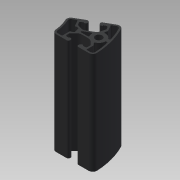
# Autodesk Inventor part: 40-4093-BLACK-FB
Saved by Autodesk Inventor 2013 (Build 170138000, 138)
## iProperties
Company: 80/20 Inc.
Created: 2014-04-23
Part Number: 40-4093-BLACK-FB
Material: Generic
Document SubType Name: Modeling
Designer: Ross Bowman
Density: 1 g/cm^3
Engineer: Ross Bowman
Catalog Web Link: 8020.net
Vendor: 80/20 Inc.
Material: 6105-T5 Aluminum
Author: Ross Bowman
Keywords: 80/20 , 8020 , T-Slot , Extrusion
Autodesk Inventor part; units mm, degrees
ref_plane "YZ Plane" through (0, 0, 0) normal (1, 0, 0) x (0, 1, 0)
ref_plane "XZ Plane" through (0, 0, 0) normal (0, 1, 0) x (-1, 0, 0)
ref_plane "XY Plane" through (0, 0, 0) normal (0, 0, 1) x (1, 0, 0)
sketch "Sketch1" plane through (0, 0, 0) normal (0, 0, 1) x (1, 0, 0)
  circle A0 centre (0, 0) radius 3.4
  arc A1 (-6.641, -0.198) -> (-5.8503, -3.149) centre (0, 0) ccw
  arc A2 (-6.5195, -4.2692) -> (-5.8503, -3.149) centre (-6.5195, -3.5092) ccw
  line L0 (-13.0965, -4.2692) -> (-6.5195, -4.2692)
  arc A3 (-13.4765, -2.851) -> (-13.0965, -4.2692) centre (-13.0965, -3.5092) ccw
  line L1 (-7.7807, 0.4375) -> (-13.4765, -2.851)
  arc A4 (-6.641, -0.198) -> (-7.7807, 0.4375) centre (-7.4007, -0.2207) ccw
  arc A5 (-1.5101, 7.5599) -> (-0.6963, 6.6074) centre (-0.776, 7.3632) ccw
  line L2 (-0.9407, 9.685) -> (-1.5101, 7.5599)
  arc A6 (-0.9407, 9.685) -> (-1.0166, 10.2617) centre (-1.6748, 9.8817) ccw
  line L3 (-4.1504, 15.6896) -> (-1.0166, 10.2617)
  arc A7 (-3.8793, 16.7237) -> (-4.1504, 15.6896) centre (-3.4922, 16.0696) ccw
  line L4 (-1.0754, 18.3829) -> (-3.8793, 16.7237)
  arc A8 (2.2157, 17.4265) -> (-1.0754, 18.3829) centre (0.1214, 16.3605) ccw
  arc A9 (7.4116, 4.4816) -> (2.2157, 17.4265) centre (-67.6148, -18.1173) ccw
  arc A10 (6.8805, 3.5283) -> (7.4116, 4.4816) centre (6.6838, 4.2624) ccw
  line L5 (6.3485, 3.3858) -> (6.8805, 3.5283)
  arc A11 (5.5204, 3.697) -> (6.3485, 3.3858) centre (6.1518, 4.1199) ccw
  arc A12 (5.5204, 3.697) -> (-0.6963, 6.6074) centre (0, 0) ccw
  arc A13 (2.7006, -6.0703) -> (6.6293, -0.4415) centre (0, 0) ccw
  arc A14 (7.1909, 0.2421) -> (6.6293, -0.4415) centre (7.3876, -0.492) ccw
  line L6 (7.7229, 0.3846) -> (7.1909, 0.2421)
  arc A15 (8.6594, -0.1754) -> (7.7229, 0.3846) centre (7.9196, -0.3495) ccw
  arc A16 (10.6314, -13.97) -> (8.6594, -0.1754) centre (-67.6148, -18.1173) ccw
  line L7 (4.2504, -9.3952) -> (4.2504, -15.6844)
  arc A17 (4.2504, -9.3952) -> (4.0278, -8.8578) centre (3.4904, -9.3952) ccw
  line L8 (2.4722, -7.3021) -> (4.0278, -8.8578)
  arc A18 (2.7006, -6.0703) -> (2.4722, -7.3021) centre (3.0096, -6.7647) ccw
  arc A19 (-17.472, -2.5855) -> (-17.8859, -2.093) centre (-18.2061, -2.7822) ccw
  line L9 (-16.4239, -6.4969) -> (-17.472, -2.5855)
  arc A20 (-16.5361, -7.1304) -> (-16.4239, -6.4969) centre (-17.158, -6.6936) ccw
  arc A21 (-18.8445, -8.5432) -> (-16.5361, -7.1304) centre (-19.3185, -5.1764) ccw
  arc A22 (-18.8445, -8.5432) -> (-19.4985, -9.2957) centre (-18.7385, -9.2957) ccw
  line L10 (-19.4985, -15.6844) -> (-19.4985, -9.2957)
  arc A23 (-26.1453, -14.3093) -> (-29.8036, -0.6665) centre (-67.6148, -18.1173) ccw
  arc A24 (-28.8231, 2.3659) -> (-29.8036, -0.6665) centre (-27.6699, 0.3183) ccw
  line L11 (-25.7487, 4.0973) -> (-28.8231, 2.3659)
  arc A25 (-24.7176, 3.8151) -> (-25.7487, 4.0973) centre (-25.3758, 3.4351) ccw
  line L12 (-21.5341, -1.6989) -> (-24.7176, 3.8151)
  arc A26 (-21.5341, -1.6989) -> (-20.5914, -2.0236) centre (-20.8759, -1.3189) ccw
  arc A27 (-17.8859, -2.093) -> (-20.5914, -2.0236) centre (-19.3185, -5.1764) ccw
  arc A28 (-3.5707, -16.5209) -> (-2.0596, -18.1044) centre (-1.9773, -16.5131) ccw
  line L13 (-2.0596, -18.1044) -> (8.2792, -18.1044)
  arc A29 (8.2792, -18.1044) -> (12.2736, -13.8932) centre (8.2792, -14.1044) ccw
  arc A30 (12.2736, -13.8932) -> (3.6826, 18.1687) centre (-67.6148, -18.1173) ccw
  arc A31 (3.6826, 18.1687) -> (-1.8822, 19.8185) centre (0.1178, 16.3544) ccw
  line L14 (-1.8822, 19.8185) -> (-10.8359, 14.6491)
  arc A32 (-10.8359, 14.6491) -> (-11.3528, 12.5222) centre (-9.969, 13.3121) ccw
  line L15 (-11.3528, 12.5222) -> (-10.8956, 11.7304)
  arc A33 (-10.8956, 11.7304) -> (-8.8041, 11.13) centre (-9.5411, 12.5058) ccw
  line L16 (-8.8041, 11.13) -> (-8.1373, 11.515)
  arc A34 (-8.1373, 11.515) -> (-7.9918, 12.0224) centre (-8.3273, 11.844) ccw
  line L17 (-7.9918, 12.0224) -> (-8.0052, 12.0476)
  arc A35 (-7.8597, 12.555) -> (-8.0052, 12.0476) centre (-7.6697, 12.226) ccw
  line L18 (-7.8597, 12.555) -> (-6.2048, 13.5105)
  arc A36 (-4.4702, 13.0457) -> (-6.2048, 13.5105) centre (-5.5699, 12.4107) ccw
  line L19 (-4.4702, 13.0457) -> (-3.2502, 10.9325)
  arc A37 (-3.1614, 10.258) -> (-3.2502, 10.9325) centre (-4.02, 10.488) ccw
  line L20 (-3.1614, 10.258) -> (-4.3643, 5.7687)
  arc A38 (-6.577, 2.8849) -> (-4.3643, 5.7687) centre (-8.9516, 6.9979) ccw
  line L21 (-6.577, 2.8849) -> (-12.4327, -0.4958)
  arc A39 (-16.0365, -0.9703) -> (-12.4327, -0.4958) centre (-14.8073, 3.6171) ccw
  line L22 (-16.0365, -0.9703) -> (-20.5258, 0.2326)
  arc A40 (-21.0655, 0.6468) -> (-20.5258, 0.2326) centre (-20.2957, 1.0912) ccw
  line L23 (-21.0655, 0.6468) -> (-22.2856, 2.76)
  arc A41 (-21.8208, 4.4946) -> (-22.2856, 2.76) centre (-21.1859, 3.3949) ccw
  line L24 (-21.8208, 4.4946) -> (-20.1659, 5.45)
  arc A42 (-19.6537, 5.3223) -> (-20.1659, 5.45) centre (-19.976, 5.121) ccw
  line L25 (-19.6537, 5.3223) -> (-19.6386, 5.2981)
  arc A43 (-19.6386, 5.2981) -> (-19.1264, 5.1704) centre (-19.3164, 5.4995) ccw
  line L26 (-19.1264, 5.1704) -> (-18.5146, 5.5237)
  arc A44 (-18.5146, 5.5237) -> (-17.9383, 7.6746) centre (-19.3019, 6.8873) ccw
  line L27 (-17.9383, 7.6746) -> (-18.3954, 8.4664)
  arc A45 (-18.3954, 8.4664) -> (-20.5464, 9.0427) centre (-19.759, 7.6791) ccw
  line L28 (-20.5464, 9.0427) -> (-29.662, 3.7798)
  arc A46 (-29.662, 3.7798) -> (-31.2941, -1.36) centre (-27.662, 0.3157) ccw
  arc A47 (-27.7815, -14.4692) -> (-31.2941, -1.36) centre (-67.6148, -18.1173) ccw
  arc A48 (-27.7815, -14.4692) -> (-23.7982, -18.1044) centre (-23.7982, -14.1044) ccw
  line L29 (-23.7982, -18.1044) -> (-13.2723, -18.1044)
  arc A49 (-13.2723, -18.1044) -> (-11.6977, -16.5298) centre (-13.2723, -16.5298) ccw
  line L30 (-11.6977, -16.5298) -> (-11.6977, -15.6155)
  arc A50 (-11.6977, -15.6155) -> (-13.2723, -14.0409) centre (-13.2723, -15.6155) ccw
  line L31 (-13.2723, -14.0409) -> (-13.9788, -14.0409)
  arc A51 (-13.9788, -14.0409) -> (-14.3585, -14.4076) centre (-13.9788, -14.4209) ccw
  line L32 (-14.3585, -14.4076) -> (-14.3595, -14.4361)
  arc A52 (-14.7392, -14.8028) -> (-14.3595, -14.4361) centre (-14.7392, -14.4229) ccw
  line L33 (-14.7392, -14.8028) -> (-16.6501, -14.8028)
  arc A53 (-17.9199, -13.533) -> (-16.6501, -14.8028) centre (-16.6501, -13.533) ccw
  line L34 (-17.9199, -13.533) -> (-17.9199, -11.0929)
  arc A54 (-17.6596, -10.4644) -> (-17.9199, -11.0929) centre (-17.031, -11.0929) ccw
  line L35 (-17.6596, -10.4644) -> (-14.3732, -7.178)
  arc A55 (-11.015, -5.787) -> (-14.3732, -7.178) centre (-11.015, -10.5362) ccw
  line L36 (-11.015, -5.787) -> (-4.2534, -5.787)
  arc A56 (-0.8952, -7.178) -> (-4.2534, -5.787) centre (-4.2534, -10.5362) ccw
  line L37 (-0.8952, -7.178) -> (2.3912, -10.4644)
  arc A57 (2.6515, -11.0929) -> (2.3912, -10.4644) centre (1.7626, -11.0929) ccw
  line L38 (2.6515, -11.0929) -> (2.6515, -13.533)
  arc A58 (1.3817, -14.8028) -> (2.6515, -13.533) centre (1.3817, -13.533) ccw
  line L39 (1.3817, -14.8028) -> (-0.5292, -14.8028)
  arc A59 (-0.9089, -14.4361) -> (-0.5292, -14.8028) centre (-0.5292, -14.4229) ccw
  line L40 (-0.9089, -14.4361) -> (-0.9099, -14.4076)
  arc A60 (-0.9099, -14.4076) -> (-1.2896, -14.0409) centre (-1.2896, -14.4209) ccw
  line L41 (-1.2896, -14.0409) -> (-2.0596, -14.0409)
  arc A61 (-2.0596, -14.0409) -> (-3.5707, -15.6066) centre (-2.01, -15.6009) ccw
  line L42 (-3.5707, -15.6066) -> (-3.5707, -16.5209)
  line L43 (5.0104, -16.4444) -> (8.2847, -16.4444)
  line L44 (-23.8052, -16.4444) -> (-20.2585, -16.4444)
  arc A62 (-26.1453, -14.3093) -> (-23.8052, -16.4444) centre (-23.8052, -14.0944) ccw
  arc A63 (8.2847, -16.4444) -> (10.6314, -13.97) centre (8.2847, -14.0944) ccw
  arc A64 (-20.2585, -16.4444) -> (-19.4985, -15.6844) centre (-20.2585, -15.6844) ccw
  arc A65 (4.2504, -15.6844) -> (5.0104, -16.4444) centre (5.0104, -15.6844) ccw
  point P0 (0, 0)
  constraints: 130 point on circle, 90 end point, 66 centre point
extrude "Extrusion1" add sketch "Sketch1" against normal blind 100
body "Solid1"
